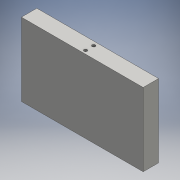
# Autodesk Inventor part: Base
Saved by Autodesk Inventor 2016 (Build 200138000, 138)
## iProperties
Created: 2016-04-04
Part Number: Base
Material: Generic
Document SubType Name: Modeling
Designer: Andres
Density: 1 g/cm^3
Appearance: Default
Author: Andres
Autodesk Inventor part; units mm, degrees
ref_plane "YZ Plane" through (0, 0, 0) normal (1, 0, 0) x (0, 1, 0)
ref_plane "XZ Plane" through (0, 0, 0) normal (0, 1, 0) x (-1, 0, 0)
ref_plane "XY Plane" through (0, 0, 0) normal (0, 0, 1) x (1, 0, 0)
sketch "Sketch1" plane through (0, 0, 0) normal (0, 1, 0) x (-1, 0, 0)
  line L0 (75, 0) -> (-75, 0)
  line L1 (-75, 0) -> (-75, -90)
  line L2 (-75, -90) -> (75, -90)
  line L3 (75, -90) -> (75, 0)
  point P0 (0, 0)
  point P1 (0, 0)
  dimension "d0" = 150
  dimension "d1" = 90
  constraints: 8 end point, 2 parallel, 1 coincident, 1 horizontal, 1 midpoint, 1 perpendicular
  measures "d0" distance of L2.end L1.end
  measures "d1" distance of L1.end L0.end
extrude "Extrusion1" add sketch "Sketch1" along normal blind 19
sketch "Sketch2" plane through (-75, 0, 0) normal (0, 0, 1) x (1, 0, 0)
  line L0 (0, 0) -> (150, 0) projected
  line L1 (150, 0) -> (150, 19) projected
  line L2 (0, 19) -> (150, 19) projected
  line L3 (0, 0) -> (0, 19) projected
  point P0 (75, 0)
  point P1 (75, 4)
  point P2 (75, 14)
  dimension "d4" = 4
  dimension "d5" = 14
  dimension "d6" = 75
  dimension "d7" = 75
  measures "d4" distance of point (75, 0) point (75, 4)
  measures "d5" distance of point (75, 14) point (75, 0)
  measures "d6" distance from line of point (75, 4) L3
  measures "d7" distance from line of point (75, 14) L3
hole "Hole1" at (0, 4, 0) at (0, 14, 0) direction (0, 0, -1) diameter 4 depth 15
sketch "Sketch3" plane through (0, 19, 0) normal (0, 1, 0) x (1, 0, 0)
  line L0 (-75, 0) -> (75, 0) projected
  line L1 (75, 0) -> (75, 90) projected
  line L2 (75, 90) -> (-75, 90) projected
  line L3 (-75, 90) -> (-75, 0) projected
  point P0 (0, 0)
  point P1 (-71.5, 87)
  point P2 (71.5, 87)
  point P3 (50, 3)
  point P4 (-50, 3)
  dimension "d15" = 143
  dimension "d16" = 3
  dimension "d17" = 3.5
  dimension "d18" = 3
  dimension "d19" = 100
  dimension "d20" = 25
  dimension "d21" = 3
  dimension "d22" = 3
  measures "d15" distance of point (71.5, 87) point (-71.5, 87)
  measures "d16" distance from line of L2 point (-71.5, 87)
  measures "d17" distance from line of point (-71.5, 87) L3
  measures "d18" distance from line of L2 point (71.5, 87)
  measures "d19" distance of point (50, 3) point (-50, 3)
  measures "d20" distance from line of L1 point (50, 3)
  measures "d21" distance from line of L0 point (-50, 3)
  measures "d22" distance from line of L0 point (50, 3)
hole "Hole2" at (-71.5, 19, -87) at (71.5, 19, -87) at (50, 19, -3) at (-50, 19, -3) direction (0, -1, 0) diameter 4 depth 15
body "Solid1"
